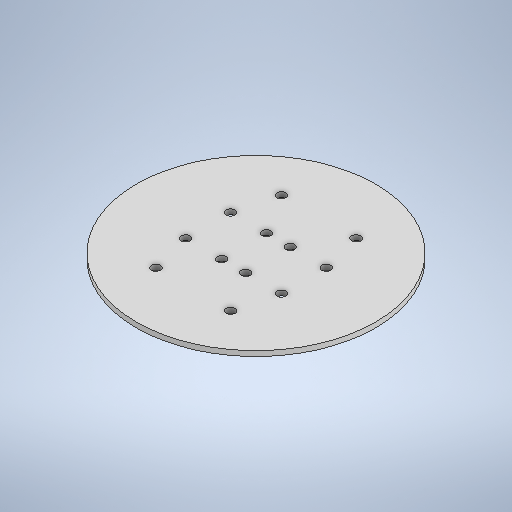
# Autodesk Inventor part: base plate
Saved by Autodesk Inventor 2025.2 (Build 292293000, 293)
## iProperties
Created: 2025-05-21
Part Number: base plate
Material: Generic
Document SubType Name: Modeling
Designer: Verchasv
Density: 1 g/cm^3
Appearance: Default
Author: Verchasv
Autodesk Inventor part; units mm, degrees
ref_plane "YZ Plane" through (0, 0, 0) normal (1, 0, 0) x (0, 1, 0)
ref_plane "XZ Plane" through (0, 0, 0) normal (0, 1, 0) x (-1, 0, 0)
ref_plane "XY Plane" through (0, 0, 0) normal (0, 0, 1) x (1, 0, 0)
sketch "Sketch1" plane through (0, 0, 0) normal (0, 1, 0) x (-1, 0, 0)
  circle A0 centre (0, 0) radius 40
  circle A1 centre (4, -7.5) radius 1.5
  circle A2 centre (16, -7.5) radius 1.5
  circle A3 centre (12.5, -21) radius 1.5
  line L0 (0, -59.049) -> (0, -66.1478)
  line L1 (48.8848, 0) -> (55.4996, 0)
  circle A4 centre (-4, -7.5) radius 1.5
  circle A5 centre (-16, -7.5) radius 1.5
  circle A6 centre (-12.5, -21) radius 1.5
  circle A7 centre (4, 7.5) radius 1.5
  circle A8 centre (16, 7.5) radius 1.5
  circle A9 centre (12.5, 21) radius 1.5
  circle A10 centre (-12.5, 21) radius 1.5
  circle A11 centre (-16, 7.5) radius 1.5
  circle A12 centre (-4, 7.5) radius 1.5
  dimension "d0" = 80
  dimension "d1" = 3
  dimension "d2" = 3
  dimension "d3" = 3
  dimension "d4" = 4
  dimension "d5" = 7.5
  dimension "d6" = 12
  dimension "d7" = 0
  dimension "d8" = 12.5
  dimension "d9" = 21
  constraints: 13 centre point, 9 symmetric about line, 4 end point, 1 coincident, 1 horizontal, 1 vertical, 9 other
  measures "d0" diameter of A0
  measures "d1" diameter of A1
  measures "d2" diameter of A2
  measures "d3" diameter of A3
  measures "d4" horizontal distance of point (0, 0) A1.centre
  measures "d5" vertical distance of point (0, 0) A1.centre
  measures "d6" distance of A1.centre A2.centre
  measures "d7" vertical distance of A2.centre A1.centre
  measures "d8" horizontal distance of point (0, 0) A3.centre
  measures "d9" vertical distance of A3.centre point (0, 0)
extrude "Extrusion1" add sketch "Sketch1" along normal blind 1.7
body "Solid1"
